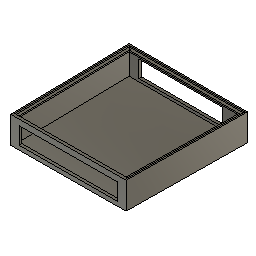
DFR0535_eclosure v10 (Autodesk Fusion 360 design; units mm, degrees)
part number: Configuração 2
Autodesk Fusion 360 part; units mm, degrees
sketch "Esboço1" plane through (0, 0, 0) normal (0, 0, 1) x (1, 0, 0)
sketch "Esboço2" plane through (0, 0, 0) normal (0, 0, 1) x (1, 0, 0)
sketch "Esboço3" plane through (0, 0, 5) normal (0, 0, 1) x (-1, 0, 0)
  line L0 (-4, -141.9652) -> (39.9838, -111.6968)
  line L1 (39.9838, -111.6968) -> (37.5306, 87.5)
  line L2 (37.5306, 87.5) -> (-45.5306, 87.5)
  line L3 (-45.5306, 87.5) -> (-47.9838, -111.6968)
  line L4 (-47.9838, -111.6968) -> (-4, -141.9652)
  line L5 (-42.9513, -109.0905) -> (-40.5796, 83.4877)
  line L6 (-40.5796, 83.4877) -> (-41.5796, 83.5)
  line L7 (-41.5796, 83.5) -> (33.5796, 83.5)
  line L8 (33.5796, 83.5) -> (32.5796, 83.4877)
  line L9 (32.5796, 83.4877) -> (34.9513, -109.0905)
  line L10 (34.9513, -109.0905) -> (-4, -135.8957)
  line L11 (-4, -135.8957) -> (-42.9513, -109.0905)
sketch "Esboço4" plane through (0, 0, 5) normal (0, 0, 1) x (-1, 0, 0)
  line L0 (-4, -61.9652) -> (39.9838, -31.6968)
  line L1 (39.9838, -31.6968) -> (37.5306, 167.5)
  line L2 (37.5306, 167.5) -> (-45.5306, 167.5)
  line L3 (-45.5306, 167.5) -> (-47.9838, -31.6968)
  line L4 (-47.9838, -31.6968) -> (-4, -61.9652)
  line L5 (-42.9513, -29.0905) -> (-40.5796, 163.4877)
  line L6 (-40.5796, 163.4877) -> (-41.5796, 163.5)
  line L7 (-41.5796, 163.5) -> (33.5796, 163.5)
  line L8 (33.5796, 163.5) -> (32.5796, 163.4877)
  line L9 (32.5796, 163.4877) -> (34.9513, -29.0905)
  line L10 (34.9513, -29.0905) -> (-4, -55.8957)
  line L11 (-4, -55.8957) -> (-42.9513, -29.0905)
  line L12 (39.9096, -25.6783) -> (38.7572, -25.6925)
  line L13 (34.9513, -29.0905) -> (37.9511, -29.0535)
  line L14 (-42.9513, -29.0905) -> (-45.9511, -29.0535)
  line L15 (37.9511, -29.0535) -> (36.4512, 56.4086)
  line L16 (-45.9511, -29.0535) -> (-44.9043, 55.94)
  line L17 (36.4512, 56.4086) -> (-44.9043, 55.94)
  line L18 (-45.9511, -29.0535) -> (37.9511, -29.0535)
  dimension "d1" = 3
  dimension "d2" = 3
  dimension "d3" = 85
  constraint coincident L1 L12.start
  constraint perpendicular L1 L12
  constraint coincident L9.end L10.start
  constraint perpendicular L9 L13
  constraint coincident L5.start L11.end
  constraint perpendicular L5 L14
  constraint perpendicular L14 L16
  measures "d1" distance of L9.end L13.end
  measures "d2" distance of L5.start L14.end
  measures "d3" distance of L14.end L16.end
extrude "Extrusão1" add sketch "Esboço4" along normal blind 1 contours L5 L16 L17 L18 | L5 L9 L17 L18 | L9 L15 L17 L18 makes body 1
sketch "Esboço5" plane through (0, 0, 6) normal (0, 0, 1) x (-1, 0, 0)
  line L0 (-45.9511, -29.0535) -> (37.9511, -29.0535)
  line L1 (37.9511, -29.0535) -> (36.4512, 56.4086)
  line L2 (36.4512, 56.4086) -> (-44.9043, 55.94)
  line L3 (-44.9043, 55.94) -> (-45.9511, -29.0535)
  line L4 (35.4687, 55.403) -> (-43.9165, 54.9457)
  line L5 (-43.9165, 54.9457) -> (-44.9387, -28.0535)
  line L6 (-44.9387, -28.0535) -> (36.9334, -28.0535)
  line L7 (36.9334, -28.0535) -> (35.4687, 55.403)
  dimension "d6" = -1
extrude "Extrusão2" add sketch "Esboço5" along normal blind 17 bodies 1
extrude "Extrusão3" add 1 faces at (-37.1119, 0.2328, 23) along direction (0, 0, 1) blind 1 on bodies 1 bodies 1
sketch "Esboço6" plane through (0, 28.0535, 0) normal (0, -1, 0) x (1, 0, 0)
  line L0 (-36.9334, 6) -> (44.9387, 6)
  line L1 (44.9387, 6) -> (44.9387, 24)
  line L2 (44.9387, 24) -> (-36.9334, 24)
  line L3 (-36.9334, 24) -> (-36.9334, 6)
  line L4 (-36.9334, 6) -> (-36.9334, 8)
  line L5 (-36.9334, 8) -> (44.9387, 8)
  line L6 (44.9387, 8) -> (44.9387, 20)
  line L7 (44.9387, 20) -> (-36.9334, 20)
  line L8 (-36.9334, 8) -> (-36.9334, 20)
  line L9 (-36.9334, 8) -> (-28.9334, 8)
  line L10 (-28.9334, 8) -> (-28.9334, 20)
  line L11 (44.9387, 8) -> (29.9387, 8)
  line L12 (29.9387, 8) -> (29.9387, 20)
  dimension "d11" = 8
  dimension "d12" = 15
  constraint coincident L0.start L3.end
  constraint coincident L3 L4.end
  constraint perpendicular L0 L4
  constraint coincident L1 L5.end
  constraint perpendicular L1 L5
  constraint coincident L1 L6.end
  constraint perpendicular L5 L6
  constraint coincident L3 L7.end
  constraint perpendicular L3 L7
  constraint perpendicular L4 L9
  constraint coincident L7 L10.end
  constraint perpendicular L7 L10
  constraint perpendicular L6 L11
  constraint coincident L7 L12.end
  constraint perpendicular L7 L12
  measures "d11" distance of L4.end L9.end
  measures "d12" distance of L5.end L11.end
extrude "Extrusão4" cut sketch "Esboço6" against normal blind 47 contours L5 L7 L10 L12 bodies 1
sketch "Esboço7" plane through (0.3179, -55.1968, 0) normal (-0.00576, 0.999983, 0) x (-0.999983, -0.00576, 0)
  line L0 (-43.5993, 6) -> (35.7872, 6)
  line L1 (35.7872, 6) -> (35.7872, 24)
  line L2 (35.7872, 24) -> (-43.5993, 24)
  line L3 (-43.5993, 24) -> (-43.5993, 6)
  line L4 (-43.5993, 6) -> (-43.5993, 8)
  line L5 (-43.5993, 8) -> (35.7872, 8)
  line L6 (-43.5993, 8) -> (-43.5993, 20)
  line L7 (-43.5993, 20) -> (-38.5993, 20)
  line L8 (-38.5993, 20) -> (-38.5993, 8)
  line L9 (-38.5993, 20) -> (-38.5993, 8)
  line L10 (35.7872, 8) -> (30.7872, 8)
  line L11 (30.7872, 8) -> (30.7872, 20)
  line L12 (30.7872, 20) -> (-38.5993, 20)
  dimension "d15" = 5
  dimension "d16" = 5
  constraint coincident L0.start L3.end
  constraint coincident L3 L4.end
  constraint perpendicular L0 L4
  constraint coincident L1 L5.end
  constraint perpendicular L1 L5
  constraint coincident L3 L6.end
  constraint perpendicular L6 L7
  constraint coincident L5 L8.end
  constraint perpendicular L5 L8
  constraint coincident L5 L10.end
  constraint perpendicular L5 L11
  constraint perpendicular L8 L12
  measures "d15" distance of L6.end L7.end
  measures "d16" distance of L5.end L10.end
extrude "Extrusão5" cut sketch "Esboço7" against normal blind 2 contours L5 L8 L9 L11 L12 bodies 1
sketch "Esboço8" plane through (-36.4298, -0.6394, 0) normal (0.999846, 0.017548, 0) x (-0.017548, 0.999846, 0)
  line L0 (-54.772, 6) -> (28.6973, 6)
  line L1 (28.6973, 6) -> (28.6973, 24)
  line L2 (28.6973, 24) -> (-54.772, 24)
  line L3 (-54.772, 24) -> (-54.772, 6)
  line L4 (-54.772, 24) -> (-54.772, 23)
  line L5 (-54.772, 23) -> (28.6973, 23)
  line L6 (28.6973, 23) -> (28.6973, 22)
  line L7 (28.6973, 22) -> (-54.772, 22)
  dimension "d19" = 1
  constraint coincident L2.end L3.start
  constraint vertical L4
  constraint coincident L1 L5.end
  constraint perpendicular L1 L5
  constraint coincident L1 L6.end
  constraint coincident L3 L7.end
  constraint perpendicular L3 L7
  measures "d19" distance of L2.end L4.end
extrude "Extrusão6" add sketch "Esboço8" along normal blind 1 contours L1 L3 L5 L6 L7 bodies 1
sketch "Esboço9" plane through (0, 28.0535, 0) normal (0, -1, 0) x (1, 0, 0)
  line L0 (-35.9332, 22) -> (-36.9334, 22)
  line L1 (-36.9334, 22) -> (-36.9334, 6)
  line L2 (-36.9334, 6) -> (44.9387, 6)
  line L3 (44.9387, 6) -> (44.9387, 24)
  line L4 (44.9387, 24) -> (-36.9334, 24)
  line L5 (-36.9334, 24) -> (-36.9334, 23)
  line L6 (-36.9334, 23) -> (-35.9332, 23)
  line L7 (-35.9332, 23) -> (-35.9332, 22)
  line L8 (29.9387, 20) -> (29.9387, 8)
  line L9 (29.9387, 8) -> (-28.9334, 8)
  line L10 (-28.9334, 8) -> (-28.9334, 20)
  line L11 (-28.9334, 20) -> (29.9387, 20)
  line L12 (-35.9332, 23) -> (-35.9332, 22)
  line L13 (-35.9332, 22) -> (44.9387, 22)
  line L14 (44.9387, 22) -> (44.9387, 23)
  line L15 (44.9387, 23) -> (-35.9332, 23)
  constraint coincident L6.end L7.start
  constraint coincident L0.start L7.end
  constraint coincident L3 L13.end
  constraint perpendicular L3 L13
  constraint coincident L3 L14.end
extrude "Extrusão7" add sketch "Esboço9" along normal blind 1 contours L3 L7 L12 L13 L14 L15 bodies 1
sketch "Esboço10" plane through (44.5864, -0.5491, 0) normal (-0.999924, 0.012314, 0) x (-0.012314, -0.999924, 0)
  line L0 (-28.6048, 23) -> (-27.6047, 23)
  line L1 (-27.6047, 23) -> (-27.6047, 22)
  line L2 (-27.6047, 22) -> (-28.6048, 22)
  line L3 (-28.6048, 22) -> (-28.6048, 6)
  line L4 (-28.6048, 6) -> (54.4007, 6)
  line L5 (54.4007, 6) -> (54.4007, 24)
  line L6 (54.4007, 24) -> (-28.6048, 24)
  line L7 (-28.6048, 24) -> (-28.6048, 23)
  line L8 (-27.6047, 23) -> (-27.6047, 22)
  line L9 (-27.6047, 22) -> (54.4007, 22)
  line L10 (54.4007, 22) -> (54.4007, 23)
  line L11 (54.4007, 23) -> (-27.6047, 23)
  constraint coincident L0.end L1.start
  constraint coincident L1.end L2.start
  constraint coincident L5 L9.end
  constraint perpendicular L5 L9
  constraint coincident L5 L10.end
  constraint perpendicular L1 L11
extrude "Extrusão8" add sketch "Esboço10" along normal blind 1 contours L1 L5 L8 L9 L10 L11 bodies 1
sketch "Esboço11" plane through (0.3179, -55.1968, 0) normal (-0.00576, 0.999983, 0) x (-0.999983, -0.00576, 0)
  line L0 (-38.5993, 8) -> (-38.5993, 20)
  line L1 (-38.5993, 20) -> (30.7872, 20)
  line L2 (30.7872, 20) -> (30.7872, 8)
  line L3 (30.7872, 8) -> (-38.5993, 8)
  line L4 (-43.5993, 6) -> (35.7872, 6)
  line L5 (35.7872, 6) -> (35.7872, 22)
  line L6 (35.7872, 22) -> (35.7872, 23)
  line L7 (35.7872, 23) -> (35.7872, 24)
  line L8 (35.7872, 24) -> (-43.5993, 24)
  line L9 (-43.5993, 24) -> (-43.5993, 23)
  line L10 (-43.5993, 23) -> (-43.5993, 22)
  line L11 (-43.5993, 22) -> (-43.5993, 6)
  line L12 (-42.6, 22) -> (-42.6, 23)
  line L13 (-42.6, 23) -> (35, 23)
  line L14 (35, 23) -> (35, 22)
  line L15 (35, 22) -> (-42.6, 22)
  constraint vertical L12
  constraint perpendicular L12 L13
  constraint perpendicular L13 L14
extrude "Extrusão9" add sketch "Esboço11" along normal blind 1 contours L12 L13 L14 L15 bodies 1
sketch "Esboço12" plane through (0, 0, 24) normal (0, 0, 1) x (-1, 0, 0)
  line L0 (35.4687, 55.403) -> (36.9334, -28.0535)
  line L1 (36.9334, -28.0535) -> (-44.9387, -28.0535)
  line L2 (-44.9387, -28.0535) -> (-43.9165, 54.9457)
  line L3 (-43.9165, 54.9457) -> (35.4687, 55.403)
  line L4 (-44.9043, 55.94) -> (-45.9511, -29.0535)
  line L5 (-45.9511, -29.0535) -> (37.9511, -29.0535)
  line L6 (37.9511, -29.0535) -> (36.4512, 56.4086)
  line L7 (36.4512, 56.4086) -> (-44.9043, 55.94)
  line L8 (-44.9387, -28.0535) -> (-44.9387, -26.0535)
  line L9 (-44.9387, -26.0535) -> (36.8983, -26.0535)
  line L10 (36.9334, -28.0535) -> (36.8983, -26.0535)
  line L11 (36.9334, -28.0535) -> (-44.9387, -28.0535)
  line L12 (-44.9387, -26.0535) -> (-42.9388, -26.0782)
  line L13 (-42.9388, -26.0782) -> (-41.9408, 54.9571)
  line L14 (36.8983, -26.0535) -> (28.8983, -26.0535)
  line L15 (28.8983, -26.0535) -> (28.4235, 56.3624)
  line L16 (-42.9388, -26.0782) -> (-42.5694, 3.9196)
  line L17 (-42.5694, 3.9196) -> (28.7234, 4.044)
  line L18 (-42.5694, 3.9196) -> (28.7238, 3.9196) construction
  line L19 (-41.9408, 54.9571) -> (28.4293, 55.3624)
  line L20 (-42.5694, 3.9196) -> (-41.9408, 54.9571)
  line L21 (28.4293, 55.3624) -> (28.7238, 3.9196)
  dimension "d28" = 2
  dimension "d29" = 2
  dimension "d30" = 8
  dimension "d31" = 30
  dimension "d32" = 0.1
  constraint coincident L1.end L2.start
  constraint perpendicular L1 L8
  constraint coincident L0 L9.end
  constraint perpendicular L8 L9
  constraint coincident L0.end L1.start
  constraint perpendicular L2 L12
  constraint coincident L3 L13.end
  constraint perpendicular L12 L13
  constraint coincident L9 L14.end
  constraint coincident L7 L15.end
  constraint perpendicular L7 L15
  constraint coincident L13 L16.end
  constraint horizontal L18
  constraint coincident L15 L19.end
  constraint coincident L3 L19.end
  measures "d28" distance of L1.end L8.end
  measures "d29" distance of L8.end L12.end
  measures "d30" distance of L9.end L14.end
  measures "d31" distance of L12.end L16.end
  measures "d32" angle of L17 L18
extrude "Extrusão1'" add sketch "Esboço12" along normal blind 1 separate body contours L0 L3 L9 L14 L15 | L0 L1 L2 L9 L10 L11 L12 L13 L14 L16 | L3 L13 L17 L19 L20 L21 | L2 L3 L9 L13 L16 L20 makes body 2 in component "Component"
move_face "Deslocar faces1" offset 8 1 faces at (18.8052, -3.961, 24.3333) on bodies 2 in component "Component"
extrude "Extrusão2'" add 2 faces at (19.385, -35.4092, 25) (-33.7668, -0.432, 25) along direction (0, 0, 1) blind 1 on bodies 2 bodies 2 in component "Component"
extrude "Extrusão10" add 1 faces at (-35.4392, -0.0967, 22.6667) along direction (0.999846, 0.017548, 0) blind 1 on bodies 1 bodies 1
extrude "Extrusão11" add 1 faces at (17.6457, 27.0535, 22.6667) along direction (0, -1, 0) blind 1 on bodies 1 bodies 1
extrude "Extrusão12" add 1 faces at (43.5816, -0.932, 22.6667) along direction (-0.999924, 0.012314, 0) blind 1 on bodies 1 bodies 1
extrude "Extrusão13" add 1 faces at (16.457, -54.1038, 22.6667) along direction (-0.00576, 0.999983, 0) blind 1 on bodies 1 bodies 1
extrude "Extrusão14" add 1 faces at (44.2572, -27.2793, 16.6667) along direction (-0.999924, 0.012314, 0) blind 1 on bodies 1 bodies 1
extrude "Extrusão15" add 1 faces at (-33.802, -55.3934, 12) along direction (-0.00576, 0.999983, 0) blind 1 on bodies 1 bodies 1
extrude "Extrusão16" add 1 faces at (-36.4451, 0.2347, 11.3333) along direction (0.999846, 0.017548, 0) blind 1 on bodies 1 bodies 1
extrude "Extrusão17" add 1 faces at (39.2719, 28.0535, 12) along direction (0, -1, 0) blind 1 on bodies 1 bodies 1
component "Component" placed x (1, 0, 0) y (0, 1, 0) z (0, 0, 1) at (0, 0, 15)
